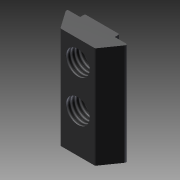
# Autodesk Inventor part: ExtrusionNutLockHNTR5-4
Saved by Autodesk Inventor 2015 SP1 (Build 190203100, 203)
## iProperties
Category: Hardware
Company: MISUMI
Created: 2015-01-29
Part Number: ExtrusionNutLockHNTR5-4
Catalog Web Link: http://us.misumi-ec.com/vona2/detail/110302247820/
Description: PACK-HNTT-Nuts for Aluminum Frames
Vendor: MISUMI
Document SubType Name: Modeling
Designer: PARTuser1
Manufacturer: MISUMI
Mass: 0.428976 g
Surface Area: 5.389 cm^2
Volume: 0.428976 cm^3
Density: 1 g/cm^3
Material: Generic
Appearance: PSOLRGB-175-175-175
Stock Number: HNTR5-4
PSOL_IDENT_0: {\\10.0.0.236\data_v8\23d-libs\misumi\metric\38_al_extrusions_blackets\nuts\pack_hntt.prj},170 {VTYP=
PSOL_IDENT_1: 3D},{NB=PACK-HNTT5-4},{LINA=PACK-HNTT5-4},{NN=PACK-HNTT},{DATE=19.11.2014 02:34:09},{GEOMDATE=31.08.
PSOL_IDENT_2: 2010 06:07:00},{VERSION=},{LINEID=10},{LINESUBID=-1},{WBVAR=M}  {NB=PACK-HNTT5-4},{LINA=PACK-HNTT5-4
PSOL_IDENT_3: },{KT=DUMMY},{PN=PACK-HNTT5-4},{TYPE=PACK-HNTT},{NO=5},{M=4},{M1=3,4,5},{A=5.800},{B=10.000},{E=3.30
PSOL_IDENT_4: 0},{T=4.100},{L=10.000}
SUPPLIER: MISUMI
ARTICLENO: PACK-HNTT5-4
BOMINFO: PACK-HNTT5-4
CREATOR: CADENAS GmbH
Title: Extrusion Nut M4 with Stop
Author: Misumi
Autodesk Inventor part; units mm, degrees
ref_plane "YZ Plane" through (0, 0, 0) normal (1, 0, 0) x (0, 1, 0)
ref_plane "XZ Plane" through (0, 0, 0) normal (0, 1, 0) x (-1, 0, 0)
ref_plane "XY Plane" through (0, 0, 0) normal (0, 0, 1) x (1, 0, 0)
sketch "Sketch_1" plane through (0, 0, 0) normal (0, 0, 1) x (1, 0, 0)
  arc A0 (-4.7999, 3.3) -> (-4.9858, 3.0264) centre (-4.7999, 3.1) ccw
  arc A1 (-4.9858, 3.0264) -> (-4.8752, 2.8208) centre (-4.056, 3.3944) ccw
  line L0 (-4.8752, 2.8208) -> (-2.9896, 0.1279)
  arc A2 (-2.9896, 0.1279) -> (-2.7438, 0) centre (-2.7438, 0.3) ccw
  line L1 (-2.7438, 0) -> (2.7438, 0)
  arc A3 (2.7438, 0) -> (2.9896, 0.1279) centre (2.7438, 0.3) ccw
  line L2 (2.9896, 0.1279) -> (4.8752, 2.8208)
  arc A4 (4.8752, 2.8208) -> (4.9858, 3.0264) centre (4.056, 3.3944) ccw
  arc A5 (4.9858, 3.0264) -> (4.7999, 3.3) centre (4.7999, 3.1) ccw
  line L3 (4.7999, 3.3) -> (2.9, 3.3)
  line L4 (2.9, 3.3) -> (2.9, 3.9)
  arc A6 (2.9, 3.9) -> (2.7, 4.1) centre (2.7, 3.9) ccw
  line L5 (2.7, 4.1) -> (-2.7, 4.1)
  arc A7 (-2.7, 4.1) -> (-2.9, 3.9) centre (-2.7, 3.9) ccw
  line L6 (-2.9, 3.9) -> (-2.9, 3.3)
  line L7 (-2.9, 3.3) -> (-4.7999, 3.3)
  constraints: 16 end point, 16 point on circle, 8 centre point
extrude "Extrusion1" add sketch "Sketch_1" along normal blind 17
sketch "Sketch3" plane through (-2.7, 4.1, 0) normal (0, 1, 0) x (1, 0, 0)
  line L0 (0, -17) -> (5.4, -17) projected
  line L1 (5.4, 0) -> (5.4, -17) projected
  line L2 (5.4, 0) -> (0, 0) projected
  circle A0 centre (2.7, -6.5) radius 2
  circle A1 centre (2.7, -13.5) radius 2
  point P0 (2.7, 0)
  dimension "d5" = 4
  dimension "d6" = 6.5
  dimension "d7" = 2.7
  dimension "d8" = 3.5
  dimension "d9" = 4
  constraints: 2 centre point, 1 vertical alignment
  measures "d5" diameter of A0
  measures "d6" distance from line of L2 A0.centre
  measures "d7" distance from line of L1 A0.centre
  measures "d8" distance from line of L0 A1.centre
  measures "d9" diameter of A1
extrude "Extrusion2" cut sketch "Sketch3" against normal up to next
thread "Thread2" size "M4x0.7" class "6H" standard "ANSI Metric M Profile" full length
thread "Thread3" size "M4x0.7" class "6H" standard "ANSI Metric M Profile" full length
body "Solid1"
